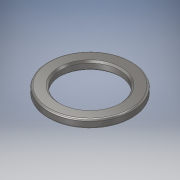
# Autodesk Inventor part: M3 Screw Washer
Saved by Autodesk Inventor 2019.2 (Build 232265000, 265)
## iProperties
Created: 2019-03-01
Part Number: M3 Screw Washer
Material: Stainless Steel
Document SubType Name: Modeling
Designer: Petar
Density: 8 g/cm^3
Appearance: Semi-Polished
Author: Petar
Autodesk Inventor part; units mm, degrees
ref_plane "YZ Plane" through (0, 0, 0) normal (1, 0, 0) x (0, 1, 0)
ref_plane "XZ Plane" through (0, 0, 0) normal (0, 1, 0) x (-1, 0, 0)
ref_plane "XY Plane" through (0, 0, 0) normal (0, 0, 1) x (1, 0, 0)
sketch "Sketch1" plane through (0, 0, 0) normal (0, 1, 0) x (-1, 0, 0)
  circle A0 centre (0, 0) radius 1.75
  circle A1 centre (0, 0) radius 2.5
  dimension "d0" = 3.5
  dimension "d1" = 5
  constraints: 2 centre point, 2 coincident
  measures "d0" diameter of A0
  measures "d1" diameter of A1
extrude "Extrusion1" add sketch "Sketch1" along normal blind 0.5
chamfer "Chamfer1" distance 0.1 angle 45 2 edges at (1.75, 0, 0) (1.75, 0.5, 0)
fillet "Fillet1" radius 0.1 2 edges at (2.5, 0.5, 0) (2.5, 0, 0)
body "Solid1"
